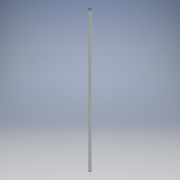
# Autodesk Inventor part: coverplate pipe
Saved by Autodesk Inventor 2018 (Build 220112000, 112)
## iProperties
Created: 2018-06-04
Part Number: coverplate pipe
Material: Generic
Document SubType Name: Modeling
Designer: John Viljoen
Density: 1 g/cm^3
Appearance: Default
Author: John Viljoen
Autodesk Inventor part; units mm, degrees
ref_plane "YZ Plane" through (0, 0, 0) normal (1, 0, 0) x (0, 1, 0)
ref_plane "XZ Plane" through (0, 0, 0) normal (0, 1, 0) x (-1, 0, 0)
ref_plane "XY Plane" through (0, 0, 0) normal (0, 0, 1) x (1, 0, 0)
sketch "Sketch1" plane through (0, 0, 0) normal (0, 0, 1) x (1, 0, 0)
  circle A0 centre (0, 0) radius 3.175
  circle A1 centre (0, 0) radius 2.675
  dimension "d0" = 6.35
  dimension "d1" = 5.35
  constraints: 2 centre point, 2 coincident
  measures "d0" diameter of A0
  measures "d1" diameter of A1
extrude "Extrusion1" add sketch "Sketch1" along normal blind 342.525
sketch "Sketch2" plane through (0, 0, 342.525) normal (0, 0, 1) x (1, 0, 0)
  circle A0 centre (0, 0) radius 2.675 projected
  circle A1 centre (0, 0) radius 3.175 projected
extrude "Extrusion2" add sketch "Sketch2" along normal blind 30.87
body "Solid1"
